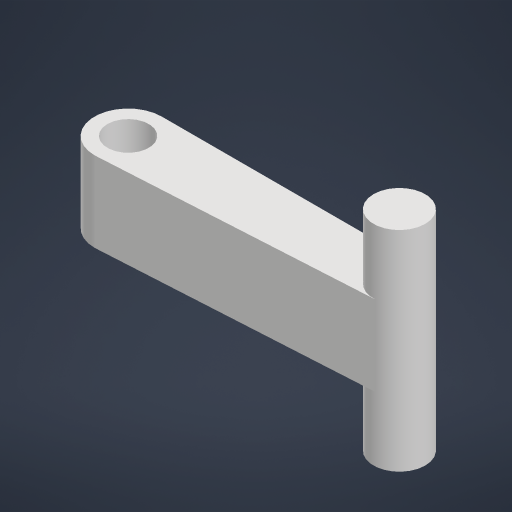
# Autodesk Inventor part: Latch
Saved by Autodesk Inventor 2024.2 (Build 282272000, 272)
## iProperties
Created: 2024-06-05
Part Number: Latch
Material: Generic
Document SubType Name: Modeling
Designer: simon
Density: 1 g/cm^3
Appearance: Default
Author: simon
Autodesk Inventor part; units mm, degrees
ref_plane "YZ Plane" through (0, 0, 0) normal (1, 0, 0) x (0, 1, 0)
ref_plane "XZ Plane" through (0, 0, 0) normal (0, 1, 0) x (-1, 0, 0)
ref_plane "XY Plane" through (0, 0, 0) normal (0, 0, 1) x (1, 0, 0)
sketch "Sketch1" plane through (0, 0, 0) normal (0, 0, 1) x (1, 0, 0)
  line L0 (0, 0) -> (25, 0)
  line L1 (25, 0) -> (25, 6.2)
  line L2 (25, 6.2) -> (0, 6.2)
  line L3 (0, 6.2) -> (0, 0)
  point P0 (25, 3.1)
  dimension "d0" = 6.2
  dimension "d1" = 25
  constraints: 8 end point, 2 parallel, 1 horizontal, 1 midpoint, 1 perpendicular
  measures "d0" distance of L2.end L0.start
  measures "d1" distance from line of point (25, 3.1) L3
extrude "Extrusion1" add sketch "Sketch1" along normal blind 5.2
sketch "Sketch2" plane through (0, 0, 0) normal (0, -1, 0) x (1, 0, 0)
  circle A0 centre (2.6, 2.6) radius 1.6
  line L0 (0, 0) -> (0, 5.2) projected
  line L1 (0, 5.2) -> (25, 5.2) projected
  dimension "d4" = 3.2
  dimension "d5" = 2.6
  dimension "d6" = 2.6
  constraints: 1 centre point
  measures "d4" diameter of A0
  measures "d5" distance from line of L0 A0.centre
  measures "d6" distance from line of L1 A0.centre
extrude "Extrusion2" cut sketch "Sketch2" against normal blind 6.5
fillet "Fillet1" radius 2.6 2 edges at (0, 3.1, 5.2) (0, 3.1, 0)
sketch "Sketch4" plane through (2.6, 6.2, 0) normal (0, 1, 0) x (1, 0, 0)
  circle A0 centre (20.4, -2) radius 2
  line L0 (22.4, 0) -> (22.4, -5.2) projected
  line L1 (22.4, 0) -> (0, 0) projected
  point P0 (-2.6, 0)
  point P1 (27.4, -4)
  dimension "d13" = 4
  dimension "d14" = 2
  dimension "d15" = 2
  constraints: 1 centre point, 1 other
  measures "d13" diameter of A0
  measures "d15" distance from line of L1 A0.centre
extrude "Extrusion4" add sketch "Sketch4" along normal blind 5 and the other way blind 11.2 contours A0
sketch "Sketch5" plane through (2.6, 6.2, 5.2) normal (0, 1, 0) x (1, 0, 0)
  arc A0 (0, 5.2) -> (0, 0) centre (0, 2.6) ccw projected
  line L0 (0, 0) -> (22.4, 1.3139)
  line L1 (22.4, 3.2) -> (22.4, 0) projected
  circle A1 centre (20.4, 3.2) radius 2 projected
  line L2 (22.4, 1.3139) -> (22.4, 0)
  line L3 (22.4, 0) -> (0, 0)
  circle A2 centre (20.4, 3.2) radius 2
  line L4 (22.4, 1.3139) -> (22.4, 3.2)
  point P0 (-2.6, 5.2)
  point P1 (20.5171, 1.2034)
  constraints: 8 end point, 2 collinear, 1 centre point, 1 coincident, 1 perpendicular, 1 point on line, 1 tangent, 1 vertical, 3 other
extrude "Extrusion5" cut sketch "Sketch5" against normal blind 6.2 contours L0 L1 L3 | A1 L1 L0
fillet "Fillet2" radius 2 1 edges at (25, 3.1, 0)
body "Solid1"
